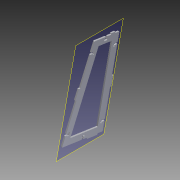
# Autodesk Inventor part: Panel_side
Saved by Autodesk Inventor 2013 (Build 170138000, 138)
## iProperties
Created: 2013-02-02
Part Number: Panel_side
Material: Aluminum 6061
Document SubType Name: Modeling
Designer: xylzlyx
Density: 1 g/cm^3
ScrewLen: 0.475 in
ScrewHoleD: 0.150 in
NutFlatsGap: 0.323 in
NutHeightGap: 0.119 in
SlotFilletRad: 0.020 in
ScrewHoleDist: 1.000 in
MetalThickness: 0.125 in
SlotWidth: 0.145 in
TabLength: 1.000 in
SlotLength: 1.020 in
SmallSlotLength: 0.395 in
SmallTabLength: 0.375 in
EdgeThickness: 0.600 in
Author: xylzlyx
Autodesk Inventor part; units mm, degrees
ref_plane "YZ Plane" through (0, 0, 0) normal (1, 0, 0) x (0, 1, 0)
ref_plane "XZ Plane" through (0, 0, 0) normal (0, 1, 0) x (-1, 0, 0)
ref_plane "XY Plane" through (0, 0, 0) normal (0, 0, 1) x (1, 0, 0)
ref_plane "Work Plane1" through (-221.4413, -90.9255, -118.1004) normal (-0.9848078, 0.1736482, 0) x (-0.1736482, -0.9848078, 0)
sketch "Sketch1" plane through (-221.4413, -90.9255, -118.1004) normal (-0.9848078, 0.1736482, 0) x (-0.1736482, -0.9848078, 0)
  line L0 (0, 0) -> (-0.5513, 3.1268) construction
  line L1 (-0.5513, 3.1268) -> (245.7896, 46.5633) construction
  line L2 (245.7896, 46.5633) -> (246.341, 43.4366) construction
  line L3 (246.341, 43.4366) -> (0, 0) construction
  line L4 (254.4978, -57.6752) -> (251.371, -58.2265) construction
  line L5 (251.371, -58.2265) -> (233.8339, 41.2312) construction
  line L6 (233.8339, 41.2312) -> (236.9607, 41.7826) construction
  line L7 (236.9607, 41.7826) -> (254.4978, -57.6752) construction
  line L8 (12.5071, 2.2053) -> (23.1628, -58.2265) construction
  line L9 (23.1628, -58.2265) -> (20.0361, -58.7779) construction
  line L10 (20.0361, -58.7779) -> (9.3803, 1.654) construction
  line L11 (9.3803, 1.654) -> (12.5071, 2.2053) construction
  line L12 (264.2669, -61.4015) -> (10.2669, -61.4015) construction
  line L13 (10.2669, -61.4015) -> (10.2669, -58.2265) construction
  line L14 (10.2669, -58.2265) -> (264.2669, -58.2265) construction
  line L15 (264.2669, -58.2265) -> (264.2669, -61.4015) construction
  line L16 (233.8339, 41.2312) -> (251.371, -58.2265)
  line L17 (251.371, -58.2265) -> (23.1628, -58.2265)
  line L18 (23.1628, -58.2265) -> (12.5071, 2.2053)
  line L19 (12.5071, 2.2053) -> (233.8339, 41.2312)
  point P0 (-127.997, 118.1004)
  constraints: 40 end point, 4 collinear, 2 horizontal, 2 vertical, 28 other
extrude "SidePanel" add sketch "Sketch1" against normal blind 3.175
fillet "CornerFillet" radius 1 4 edges at (-263.5281, -338.7532, -176.327) (-260.4828, -321.4826, -76.8692) (-223.9001, -114.0121, -176.327) (-222.0498, -103.5182, -115.8951)
sketch "ScrewSketch" plane through (-221.4413, -90.9255, -118.1004) normal (-0.9848078, 0.1736482, 0) x (0, 0, 1)
  line L0 (-57.0529, -251.164) -> (40.2464, -234.0076) projected
  line L1 (41.0576, -232.8491) -> (2.379, -13.4919) projected
  line L2 (-61.4015, -11.2669) -> (-61.4015, -263.2669) projected
  line L3 (-58.2265, -250.1792) -> (-58.2265, -24.0019) projected
  line L4 (-61.4015, -226.6779) -> (-49.3365, -226.6779)
  line L5 (-61.4015, -222.8806) -> (-49.3365, -222.8806)
  line L6 (-61.4015, -222.8806) -> (-61.4015, -226.6779)
  line L7 (-49.3365, -226.6779) -> (-49.3365, -222.8806)
  line L8 (-61.4015, -47.5033) -> (-49.3365, -47.5033)
  line L9 (-49.3365, -47.5033) -> (-49.3365, -51.3006)
  line L10 (-49.3365, -51.3006) -> (-61.4015, -51.3006)
  line L11 (-61.4015, -51.3006) -> (-61.4015, -47.5033)
  line L12 (3.3004, -0.4335) -> (46.3897, -244.8048) projected
  line L13 (-2.295, -38.1799) -> (9.5867, -36.0848)
  line L14 (-2.295, -38.1799) -> (-1.6356, -41.9195)
  line L15 (-1.6356, -41.9195) -> (10.2461, -39.8245)
  line L16 (10.2461, -39.8245) -> (9.5867, -36.0848)
  line L17 (28.2217, -211.2485) -> (40.1034, -209.1535)
  line L18 (28.2217, -211.2485) -> (27.5623, -207.5089)
  line L19 (27.5623, -207.5089) -> (39.444, -205.4138)
  line L20 (39.444, -205.4138) -> (40.1034, -209.1535)
  line L21 (40.7978, -237.1343) -> (-56.6904, -254.3241) projected
  line L22 (0.6692, -9.5539) -> (-57.2417, -19.7652) projected
  line L23 (-49.3365, -228.875) -> (-49.3365, -220.6835)
  line L24 (-49.3365, -220.6835) -> (-52.3687, -220.6835)
  line L25 (-49.3365, -228.875) -> (-52.3687, -228.875)
  line L26 (-52.3687, -228.875) -> (-52.3687, -220.6835)
  line L27 (-49.3365, -45.3062) -> (-49.3365, -53.4977)
  line L28 (-49.3365, -53.4977) -> (-52.3687, -53.4977)
  line L29 (-52.3687, -53.4977) -> (-52.3687, -45.3062)
  line L30 (-52.3687, -45.3062) -> (-49.3365, -45.3062)
  line L31 (-1.2541, -44.0832) -> (-2.6765, -36.0162)
  line L32 (-1.2541, -44.0832) -> (1.732, -43.5567)
  line L33 (1.732, -43.5567) -> (0.3095, -35.4897)
  line L34 (0.3095, -35.4897) -> (-2.6765, -36.0162)
  line L35 (28.6032, -213.4122) -> (27.1808, -205.3452)
  line L36 (27.1808, -205.3452) -> (30.1668, -204.8187)
  line L37 (30.1668, -204.8187) -> (31.5893, -212.8857)
  line L38 (31.5893, -212.8857) -> (28.6032, -213.4122)
  line L39 (-6.0765, -245.3995) -> (-8.1716, -233.5178)
  line L40 (-11.9112, -234.1772) -> (-9.8161, -246.0589)
  line L41 (-8.1716, -233.5178) -> (-11.9112, -234.1772)
  line L42 (-6.0765, -245.3995) -> (-9.8161, -246.0589)
  line L43 (-14.0749, -234.5587) -> (-6.0079, -233.1363)
  line L44 (-13.5484, -237.5448) -> (-14.0749, -234.5587)
  line L45 (-13.5484, -237.5448) -> (-5.4813, -236.1223)
  line L46 (-5.4813, -236.1223) -> (-6.0079, -233.1363)
  line L47 (-26.4165, -14.3299) -> (-24.3214, -26.2116)
  line L48 (-24.3214, -26.2116) -> (-28.061, -26.871)
  line L49 (-28.061, -26.871) -> (-30.1561, -14.9893)
  line L50 (-30.1561, -14.9893) -> (-26.4165, -14.3299)
  line L51 (-30.2247, -27.2525) -> (-22.1577, -25.8301)
  line L52 (-22.1577, -25.8301) -> (-22.6842, -22.844)
  line L53 (-22.6842, -22.844) -> (-30.7513, -24.2664)
  line L54 (-30.7513, -24.2664) -> (-30.2247, -27.2525)
  line L55 (-61.4015, -224.7792) -> (-49.3365, -224.7792) construction
  line L56 (-61.4015, -49.4019) -> (-49.3365, -49.4019) construction
  line L57 (9.9164, -37.9547) -> (-1.9653, -40.0497) construction
  line L58 (39.7737, -207.2836) -> (27.892, -209.3787) construction
  point P0 (-7.9463, -245.7292)
  point P1 (-10.0414, -233.8475)
  point P2 (-28.2863, -14.6596)
  point P3 (-26.1912, -26.5413)
  dimension "d7" = 12.065
  dimension "d8" = 3.7973
  dimension "d10" = 12.065
  dimension "d11" = 3.7973
  dimension "d14" = 12.065
  dimension "d17" = 3.7973
  dimension "d18" = 12.065
  dimension "d20" = 3.7973
  dimension "d21" = 8.1915
  dimension "d22" = 3.0321
  dimension "d23" = 8.1915
  dimension "d24" = 3.0321
  dimension "d25" = 8.1915
  dimension "d26" = 3.0321
  dimension "d27" = 8.1915
  dimension "d28" = 3.0321
  dimension "d29" = 12.065
  dimension "d30" = 3.7973
  dimension "d31" = 8.1915
  dimension "d32" = 3.0321
  dimension "d33" = 3.7973
  dimension "d34" = 12.065
  dimension "d35" = 8.1915
  dimension "d36" = 3.0321
  dimension "d40" = 25.4
  dimension "d41" = 25.4
  dimension "d42" = 25.4
  dimension "d43" = 25.4
  constraints: 104 end point, 39 parallel, 16 midpoint, 9 collinear, 6 perpendicular, 6 point on line
  measures "d7" distance of L4.start L4.end
  measures "d8" distance between parallel lines of L4 L5
  measures "d10" distance of L8.start L8.end
  measures "d11" distance of L10.end L8.start
  measures "d14" distance of L13.start L13.end
  measures "d17" distance between parallel lines of L13 L15
  measures "d18" distance of L17.start L17.end
  measures "d20" distance of L19.end L17.end
  measures "d21" distance of L23.start L23.end
  measures "d22" distance of L23.end L24.end
  measures "d23" distance of L27.start L27.end
  measures "d24" distance of L27.end L28.end
  measures "d25" distance of L31.start L31.end
  measures "d26" distance of L31.start L32.end
  measures "d27" distance of L35.start L35.end
  measures "d28" distance of L35.end L36.end
  measures "d29" distance of L39.start L39.end
  measures "d30" distance of L39.end L40.start
  measures "d31" distance of L43.start L43.end
  measures "d32" distance of L44.start L43.start
  measures "d33" distance of L49.end L47.start
  measures "d34" distance of L48.end L49.end
  measures "d35" distance of L51.start L51.end
  measures "d36" distance of L51.end L52.end
  measures "d40" vertical distance of L55.start L3.start
  measures "d41" vertical distance of L3.end L56.start
  measures "d42" distance from line of L1.end L57
  measures "d43" distance from line of L1.start L58
extrude "ScrewSlots" cut sketch "ScrewSketch" against normal blind 25.4 contours L40 L45 L39 L0 | L0 L39 L21 L40 | L45 L44 L43 L40 | L40 L41 L39 L45 | L39 L43 L46 L45 | L17 L37 L19 L1 | L1 L19 L12 L17 | L37 L38 L35 L17 | L17 L18 L19 L37 | L15 L33 L13 L1 | L1 L13 L12 L15 | L19 L35 L36 L37 | L33 L32 L31 L15 | L15 L14 L13 L33 | L13 L31 L34 L33 | L8 L3 L10 L2 | L8 L29 L10 L3 | L5 L3 L4 L2 | L29 L30 L27 L8 | L8 L9 L10 L29 | L5 L26 L4 L3 | L10 L27 L28 L29 | L26 L24 L23 L5 | L5 L7 L4 L26 | L4 L23 L25 L26 | L47 L53 L49 L22 | L53 L52 L51 L47 | L47 L48 L49 L53 | L49 L51 L54 L53
fillet "SlotFillets" radius 0.5 48 edges at (-261.9482, -329.7932, -124.7283) (-260.9464, -324.112, -125.7455) (-262.0627, -330.4426, -128.4679) (-261.0609, -324.7613, -129.4851) (-261.1272, -325.1371, -131.6488) (-260.6087, -322.1964, -132.1754) (-260.3617, -320.7956, -124.1083) (-260.8802, -323.7362, -123.5818) (-256.4695, -298.7218, -86.8927) (-256.8452, -300.8526, -86.5112) (-256.9366, -301.3712, -89.4972) (-255.5358, -293.4267, -90.9197) (-255.4443, -292.9081, -87.9336) (-255.8201, -295.039, -87.5521) (-256.2928, -297.72, -81.1238) (-255.6434, -294.0372, -81.7832) (-259.6217, -316.599, -167.437) (-259.6217, -316.599, -170.4691) (-259.2402, -314.4353, -170.4691) (-259.2402, -314.4353, -176.327) (-258.5808, -310.6957, -176.327) (-258.5808, -310.6957, -170.4691) (-258.1992, -308.5319, -170.4691) (-258.1992, -308.5319, -167.437) (-229.1677, -143.8861, -167.437) (-229.1677, -143.8861, -170.4691) (-228.7862, -141.7223, -170.4691) (-228.7862, -141.7223, -176.327) (-228.1268, -137.9827, -176.327) (-228.1268, -137.9827, -170.4691) (-227.7453, -135.819, -170.4691) (-227.7453, -135.819, -167.437) (-224.6103, -118.0396, -148.3252) (-224.3633, -116.6388, -140.2581) (-223.8448, -113.6981, -140.7846) (-223.911, -114.0738, -142.9484) (-224.0255, -114.7232, -146.688) (-224.0918, -115.0989, -148.8517) (-223.0238, -109.0419, -147.7052) (-222.9093, -108.3926, -143.9656) (-226.1321, -126.6701, -120.777) (-227.4415, -134.0961, -116.3685) (-227.5329, -134.6146, -119.3545) (-226.0407, -126.1516, -117.7909) (-226.2398, -127.2807, -111.6405) (-226.8891, -130.9635, -110.9811) (-226.4164, -128.2825, -117.4094) (-227.0658, -131.9653, -116.75)
sketch "TopTabSketch" plane through (-260.0573, -309.9276, -176.327) normal (0, 0, -1) x (-0.9848078, 0.1736482, 0)
  line L0 (0, 72.59) -> (-3.175, 72.59)
  line L1 (-3.175, 72.59) -> (-3.175, 97.99)
  line L2 (-3.175, 97.99) -> (0, 97.99)
  line L3 (0, 97.99) -> (0, 72.59)
  line L4 (0.254, 72.836) -> (0.254, 97.744) projected
  line L5 (-2.929, 72.336) -> (-0.246, 72.336) projected
  point P0 (-3.175, -27.7987)
  point P1 (0, 85.29)
  point P2 (0.254, 85.29)
  point P3 (-1.5875, 72.59)
  point P4 (-1.5875, 72.336)
  dimension "d44" = 25.4
  constraints: 8 end point, 4 midpoint, 2 parallel, 2 vertical alignment, 1 horizontal, 1 horizontal alignment, 1 perpendicular
  measures "d44" distance of L0.end L1.end
extrude "TopTab" add sketch "TopTabSketch" along normal blind 3.175
fillet "TopTabFillet" radius 0.5 4 edges at (-245.8888, -238.7161, -179.502) (-245.8888, -238.7161, -176.327) (-241.4782, -213.7019, -179.502) (-241.4782, -213.7019, -176.327)
sketch "BottomTabSketch" plane through (-257.1213, -293.2766, -81.87) normal (0.0301537, 0.1710101, 0.9848078) x (0.9848078, -0.1736482, 0)
  line L0 (3.175, 96.2719) -> (0, 96.2719)
  line L1 (0, 96.2719) -> (0, 70.8719)
  line L2 (0, 70.8719) -> (3.175, 70.8719)
  line L3 (3.175, 70.8719) -> (3.175, 96.2719)
  line L4 (2.929, 96.5259) -> (0.246, 96.5259) projected
  line L5 (-0.254, 96.0259) -> (-0.254, 71.1179) projected
  point P0 (3.175, 167.1439)
  point P1 (202.2881, 314.187)
  point P2 (0, 83.5719)
  point P3 (-0.254, 83.5719)
  point P4 (1.5875, 96.2719)
  point P5 (1.5875, 96.5259)
  dimension "d50" = 25.4
  constraints: 8 end point, 4 midpoint, 2 parallel, 2 vertical alignment, 1 horizontal, 1 horizontal alignment, 1 perpendicular
  measures "d50" distance of L2.end L0.start
extrude "BottomTab" add sketch "BottomTabSketch" along normal blind 3.175
fillet "BottomTabFillet" radius 0.5 4 edges at (-239.0945, -200.1833, -98.5875) (-238.9987, -199.6404, -95.4607) (-243.3424, -224.2745, -91.0501) (-243.4381, -224.8174, -94.1768)
sketch "BackTabSketch" plane through (-265.0555, -338.2738, -175.1533) normal (-0.1710101, -0.9698463, 0.1736482) x (0.9848078, -0.1736482, 0)
  line L0 (0, 11.3563) -> (3.175, 11.3563)
  line L1 (3.175, 11.3563) -> (3.175, 36.7563)
  line L2 (3.175, 36.7563) -> (0, 36.7563)
  line L3 (0, 36.7563) -> (0, 11.3563)
  line L4 (2.929, 37.0103) -> (0.246, 37.0103) projected
  line L5 (-0.254, 36.5103) -> (-0.254, 11.6023) projected
  point P0 (0, 0)
  point P1 (202.2881, 238.333)
  point P2 (-0.254, 24.0563)
  point P3 (0, 24.0563)
  point P4 (1.5875, 36.7563)
  point P5 (1.5875, 37.0103)
  dimension "d56" = 25.4
  constraints: 8 end point, 4 midpoint, 2 parallel, 2 vertical alignment, 1 horizontal, 1 horizontal alignment, 1 perpendicular
  measures "d56" distance of L0.end L1.end
extrude "BackTab" add sketch "BackTabSketch" along normal blind 3.175
fillet "BackTabFillet" radius 0.5 4 edges at (-262.3838, -332.2637, -138.9555) (-262.9268, -335.343, -138.4042) (-263.6927, -339.6867, -163.4183) (-263.1497, -336.6074, -163.9696)
sketch "FrontTabSketch" plane through (-225.4382, -113.5929, -175.5006) normal (0.1710101, 0.9698463, -0.1736482) x (0.9848078, -0.1736482, 0)
  line L0 (3.175, -10.1593) -> (0, -10.1593)
  line L1 (0, -10.1593) -> (0, -19.6843)
  line L2 (0, -19.6843) -> (3.175, -19.6843)
  line L3 (3.175, -19.6843) -> (3.175, -10.1593)
  line L4 (2.929, -9.9053) -> (0.246, -9.9053) projected
  line L5 (-0.254, -10.4053) -> (-0.254, -19.4383) projected
  point P0 (3.175, 0)
  point P1 (202.2881, -199.0577)
  point P2 (0, -14.9218)
  point P3 (-0.254, -14.9218)
  point P4 (1.5875, -10.1593)
  point P5 (1.5875, -9.9053)
  dimension "d61" = 9.525
  constraints: 8 end point, 4 midpoint, 2 parallel, 2 vertical alignment, 1 horizontal, 1 horizontal alignment, 1 perpendicular
  measures "d61" distance of L2.end L0.start
extrude "FrontTab" add sketch "FrontTabSketch" along normal blind 3.175
fillet "FrontTabFillet" radius 0.5 4 edges at (-223.5685, -112.1312, -165.4957) (-223.0255, -109.052, -166.047) (-222.7383, -107.4231, -156.6667) (-223.2813, -110.5023, -156.1154)
sketch "Sketch7" plane through (-221.4413, -90.9255, -118.1004) normal (-0.9848078, 0.1736482, 0) x (0, 0, 1)
  line L0 (-47.8876, -21.3398) -> (-57.4002, -23.0171) projected
  line L1 (-58.2265, -24.0019) -> (-58.2265, -47.0033) projected
  line L2 (-58.2265, -227.1779) -> (-58.2265, -250.1792) projected
  line L3 (-57.0529, -251.164) -> (-46.3616, -249.2789) projected
  line L4 (-6.1355, -242.1859) -> (40.2464, -234.0076) projected
  line L5 (41.0576, -232.8491) -> (37.0634, -210.1972) projected
  line L6 (6.3731, -36.1438) -> (2.379, -13.4919) projected
  line L7 (1.2205, -12.6807) -> (-25.3727, -17.3698) projected
  line L8 (-42.9865, -233.2087) -> (23.5764, -221.4718)
  line L9 (23.5764, -221.4718) -> (-10.1567, -30.1619)
  line L10 (-10.1567, -30.1619) -> (-42.9865, -35.9507)
  line L11 (-42.9865, -35.9507) -> (-42.9865, -233.2087)
  point P0 (118.1004, 127.997)
  dimension "d66" = 15.24
  dimension "d67" = 15.24
  dimension "d68" = 15.24
  dimension "d69" = 15.24
  dimension "d70" = 15.24
  dimension "d71" = 15.24
  dimension "d72" = 15.24
  dimension "d73" = 15.24
  constraints: 8 end point
  measures "d66" distance from line of L8.start L2
  measures "d67" distance from line of L3 L8.start
  measures "d68" distance from line of L4 L8.end
  measures "d69" distance from line of L5 L8.end
  measures "d70" distance from line of L6 L9.end
  measures "d71" distance from line of L7 L9.end
  measures "d72" distance from line of L1 L10.end
  measures "d73" distance from line of L0 L10.end
extrude "InsideGap" cut sketch "Sketch7" against normal blind 3.175
fillet "InsideGapFillet" radius 0.5 4 edges at (-260.3742, -320.8668, -161.087) (-258.3361, -309.3083, -94.5241) (-225.1155, -120.9048, -128.2572) (-226.1207, -126.6057, -161.087)
equation "\"d7\" = ScrewLen"
equation "\"d8\" = ScrewHoleD"
equation "\"d10\" = ScrewLen"
equation "\"d11\" = ScrewHoleD"
equation "\"d14\" = ScrewLen"
equation "\"d17\" = ScrewHoleD"
equation "\"d18\" = ScrewLen"
equation "\"d20\" = ScrewHoleD"
equation "\"d21\" = NutFlatsGap"
equation "\"d22\" = NutHeightGap"
equation "\"d23\" = NutFlatsGap"
equation "\"d24\" = NutHeightGap"
equation "\"d25\" = NutFlatsGap"
equation "\"d26\" = NutHeightGap"
equation "\"d27\" = NutFlatsGap"
equation "\"d28\" = NutHeightGap"
equation "\"d29\" = ScrewLen"
equation "\"d30\" = ScrewHoleD"
equation "\"d31\" = NutFlatsGap"
equation "\"d32\" = NutHeightGap"
equation "\"d33\" = ScrewHoleD"
equation "\"d34\" = ScrewLen"
equation "\"d35\" = NutFlatsGap"
equation "\"d36\" = NutHeightGap"
equation "\"ScrewLen\" = 12.065"
equation "\"ScrewHoleD\" = 3.7973"
equation "\"NutFlatsGap\" = 8.1915"
equation "\"NutHeightGap\" = 3.03212"
equation "\"SlotFilletRad\" = 0.5"
equation "\"ScrewHoleDist\" = 25.4"
equation "\"MetalThickness\" = 3.175"
equation "\"SlotWidth\" = 3.683"
equation "\"TabLength\" = 25.4"
equation "\"SlotLength\" = 25.908"
equation "\"SmallSlotLength\" = 10.033"
equation "\"SmallTabLength\" = 9.525"
equation "\"WasherHeight\" = 1.27"
equation "\"EdgeThickness\" = 15.24"
body "Solid1"
